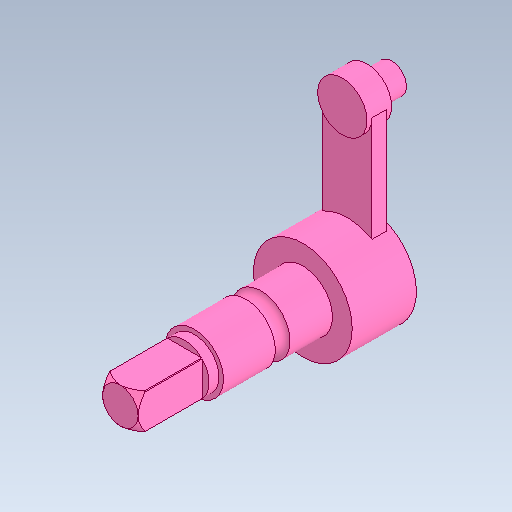
# Autodesk Inventor part: Crank
Saved by Autodesk Inventor 2020.5 (Build 245400000, 400)
## iProperties
Created: 2018-04-07
Part Number: Crank
Document SubType Name: Modeling
Designer: Administrator
Density: 7.85 g/cm^3
Mass: 64.2078 g
Surface Area: 44.7148 cm^2
Volume: 8.17933 cm^3
Material: Acero, carbono
Appearance: Pink
Author: Administrator
Autodesk Inventor part; units mm, degrees
ref_plane "YZ Plane" through (0, 0, 0) normal (1, 0, 0) x (0, 1, 0)
ref_plane "XZ Plane" through (0, 0, 0) normal (0, 1, 0) x (-1, 0, 0)
ref_plane "XY Plane" through (0, 0, 0) normal (0, 0, 1) x (1, 0, 0)
sketch "Sketch1" plane through (0, 0, 0) normal (0, 0, 1) x (1, 0, 0)
  circle A0 centre (0, 0) radius 6
  arc A1 (-5, 8.6603) -> (5, 8.6603) centre (0, 0) ccw
  line L0 (0, 0) -> (0, 30) construction
  circle A2 centre (0, 30) radius 3 construction
  arc A3 (5, 30) -> (-5, 30) centre (0, 30) ccw
  line L1 (-5, 8.6603) -> (-5, 30)
  line L2 (5, 8.6603) -> (5, 30)
  dimension "d0" = 30
  dimension "d1" = 6
  dimension "d2" = 10
  dimension "d3" = 12
  dimension "d4" = 20
  constraints: 6 end point, 4 centre point, 4 point on circle, 3 coincident, 2 symmetric about line, 1 parallel, 1 tangent, 1 vertical, 1 other
  measures "d0" distance of L0.start L0.end
  measures "d1" diameter of A2
  measures "d2" diameter of A3
  measures "d3" diameter of A0
  measures "d4" diameter of A1
extrude "Extrusion1" add sketch "Sketch1" along normal mid plane 5
sketch "Sketch2" plane through (0, 0, -2.5) normal (0, 0, -1) x (-1, 0, 0)
  arc A0 (-5, 8.6603) -> (5, 8.6603) centre (0, 0) ccw projected
  line L0 (5, 30) -> (5, 8.6603) projected
  arc A1 (5, 30) -> (-5, 30) centre (0, 30) ccw projected
  line L1 (-5, 8.6603) -> (-5, 30) projected
  circle A2 centre (0, 0) radius 10
  circle A3 centre (0, 30) radius 5
  constraints: 2 centre point, 2 coincident, 2 concentric
extrude "Extrusion2" cut sketch "Sketch2" against normal blind 1 contours L1 A3 L0 A2
mirror "Mirror1" about plane through (0, 0, 0) normal (0, 0, 1) of "Extrusion2"
sketch "Sketch3" plane through (0, 0, 2.5) normal (0, 0, 1) x (1, 0, 0)
  circle A0 centre (0, 0) radius 6 projected
  circle A1 centre (0, 0) radius 10 projected
extrude "Extrusion3" add sketch "Sketch3" along normal blind 3
sketch "Sketch4" plane through (0, 0, -2.5) normal (0, 0, -1) x (-1, 0, 0)
  circle A0 centre (0, 0) radius 6 projected
  circle A1 centre (0, 0) radius 5.9
  dimension "d12" = 0.1
  constraints: 1 centre point
  measures "d12" radial gap between concentric circles of A0 A1
extrude "Extrusion4" add sketch "Sketch4" against normal blind 35 contours A1
sketch "Sketch5" plane through (0, 30, -2.5) normal (0, 0, -1) x (-1, 0, 0)
  circle A0 centre (0, 0) radius 5 projected
  circle A1 centre (0, 0) radius 3
  dimension "d15" = 6
  constraints: 1 centre point
  measures "d15" diameter of A1
extrude "Extrusion5" add sketch "Sketch5" along normal blind 5 contours A1
sketch "Sketch6" plane through (0, 0, 32.5) normal (0, 0, 1) x (1, 0, 0)
  circle A0 centre (0, 0) radius 5.9 projected
  circle A1 centre (0, 0) radius 5
  dimension "d18" = 10
  constraints: 1 centre point
  measures "d18" diameter of A1
extrude "Extrusion6" add sketch "Sketch6" along normal blind 15 contours A1
chamfer "Chamfer1" distance 1.4 angle 45 1 edges at (-5, 0, 47.5)
sketch "Sketch7" plane through (0, 0, 47.5) normal (0, 0, 1) x (1, 0, 0)
  circle A0 centre (0, 0) radius 3.6 projected
  line L0 (3.6, 3.6) -> (3.6, -3.6)
  line L1 (3.6, -3.6) -> (-3.6, -3.6)
  line L2 (-3.6, -3.6) -> (-3.6, 3.6)
  line L3 (-3.6, 3.6) -> (3.6, 3.6)
  circle A1 centre (0, 0) radius 7.459
  point P0 (0, 3.6)
  constraints: 8 end point, 2 coincident, 1 centre point, 1 midpoint, 1 vertical alignment, 10 other
extrude "Extrusion7" cut sketch "Sketch7" against normal blind 13
sketch "Sketch8" plane through (0, 0, 0) normal (0, 1, 0) x (-1, 0, 0)
  point P0 (0, 0)
sketch "Sketch9" plane through (0, 0, 0) normal (1, 0, 0) x (0, 1, 0)
  line L0 (-5.9, 32.5) -> (5.9, 32.5) projected
  line L1 (-5.9, -2.5) -> (-5.9, 32.5) projected
  line L2 (5.9, -2.5) -> (5.9, 32.5) projected
  line L3 (-5, 32.5) -> (5, 32.5) projected
  line L4 (0, 32.5) -> (0, 20.5) construction
  line L5 (0, 20.5) -> (-5.9, 20.5) construction
  circle A0 centre (-5.9, 20.5) radius 1.5
  point P0 (0, 0)
  dimension "d26" = 3
  dimension "d27" = 12
  constraints: 4 end point, 1 centre point, 1 coincident, 1 midpoint, 1 perpendicular, 1 point on line, 1 vertical
  measures "d26" diameter of A0
  measures "d27" distance of L4.start L4.end
revolve "Revolution1" cut sketch "Sketch9" angle 360 about axis through (0, 0, 32.5) along (0, 0, -1)
sketch "Sketch10" plane through (0, 0, 5.5) normal (0, 0, 1) x (1, 0, 0)
  circle A0 centre (0, 0) radius 6 projected
  circle A1 centre (0, 0) radius 10 projected
extrude "Extrusion8" add sketch "Sketch10" along normal blind 5
body "Solid1"
